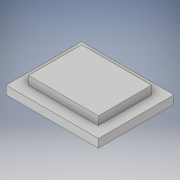
# Autodesk Inventor part: Colorimeter_Seal_Detector
Saved by Autodesk Inventor 2019 (Build 230136000, 136)
## iProperties
Created: 2019-04-03
Part Number: Colorimeter_Seal_Detector
Material: Generic
Document SubType Name: Modeling
Designer: Hansen
Density: 1 g/cm^3
Appearance: Default
Author: Hansen
Autodesk Inventor part; units mm, degrees
ref_plane "YZ Plane" through (0, 0, 0) normal (1, 0, 0) x (0, 1, 0)
ref_plane "XZ Plane" through (0, 0, 0) normal (0, 1, 0) x (-1, 0, 0)
ref_plane "XY Plane" through (0, 0, 0) normal (0, 0, 1) x (1, 0, 0)
sketch "Sketch1" plane through (0, 0, 0) normal (0, 1, 0) x (-1, 0, 0)
  line L0 (-8.25, 6.75) -> (8.25, 6.75)
  line L1 (8.25, 6.75) -> (8.25, -6.75)
  line L2 (8.25, -6.75) -> (-8.25, -6.75)
  line L3 (-8.25, -6.75) -> (-8.25, 6.75)
  line L4 (-8.25, 6.75) -> (8.25, -6.75) construction
  line L5 (8.25, 6.75) -> (-8.25, -6.75) construction
  point P0 (0, 0)
  dimension "d0" = 16.5
  dimension "d1" = 13.5
  constraints: 12 end point, 2 midpoint, 2 parallel, 1 horizontal, 1 perpendicular
  measures "d0" distance of L0.start L0.end
  measures "d1" distance of L0.end L1.end
extrude "Extrusion1" add sketch "Sketch1" along normal blind 1.5
sketch "Sketch2" plane through (0, 1.5, 0) normal (0, 1, 0) x (1, 0, 0)
  line L0 (6.25, -4.75) -> (-6.25, -4.75)
  line L1 (-6.25, -4.75) -> (-6.25, 4.75)
  line L2 (-6.25, 4.75) -> (6.25, 4.75)
  line L3 (6.25, 4.75) -> (6.25, -4.75)
  line L4 (6.25, -4.75) -> (-6.25, 4.75) construction
  line L5 (-6.25, -4.75) -> (6.25, 4.75) construction
  line L6 (-8.25, 6.75) -> (-8.25, -6.75) projected
  line L7 (-8.25, -6.75) -> (8.25, -6.75) projected
  point P0 (0, 0)
  dimension "d4" = 2
  dimension "d5" = 2
  constraints: 12 end point, 2 midpoint, 2 parallel, 1 horizontal, 1 perpendicular
  measures "d4" distance between parallel lines of L1 L6
  measures "d5" distance between parallel lines of L7 L0
extrude "Extrusion2" add sketch "Sketch2" along normal blind 1.5
equation "\"d5\" = d4"
body "Solid1"
